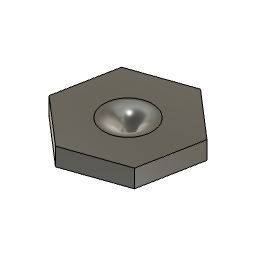
HandBaseP2 v2 (Autodesk Fusion 360 design; units mm, degrees)
Autodesk Fusion 360 part; units mm, degrees
sketch "Sketch1" plane through (0, 0, 0) normal (0, 0, 1) x (1, 0, 0)
  line L0 (9.2315, 7.937) -> (25.5856, 13.6416)
  line L1 (25.5856, 13.6416) -> (38.703, 2.3308)
  line L2 (38.703, 2.3308) -> (35.4663, -14.6846)
  line L3 (35.4663, -14.6846) -> (19.1122, -20.3892)
  line L4 (19.1122, -20.3892) -> (5.9948, -9.0784)
  line L5 (5.9948, -9.0784) -> (9.2315, 7.937)
  circle A0 centre (22.3489, -3.3738) radius 1.75
  dimension "d1" = 120
  dimension "d2" = 120
  dimension "d3" = 120
  dimension "d4" = 120
  dimension "d5" = 120
  dimension "d6" = 30
  dimension "d7" = 30
  dimension "d8" = 30
  dimension "d9" = 3.5
  constraint equal L4 L5
  measures "d1" angle of L4 L5
  measures "d2" angle of L0 L5
  measures "d3" angle of L0 L1
  measures "d4" angle of L1 L2
  measures "d5" angle of L2 L3
  measures "d6" distance of L2 L5
  measures "d7" distance of L1 L4
  measures "d8" distance of L0 L3
  measures "d9" diameter of A0
extrude "Extrude1" add sketch "Sketch1" along normal blind 5
fillet "Fillet1" radius 5 1 edges at (20.7173, -2.741, 5)
